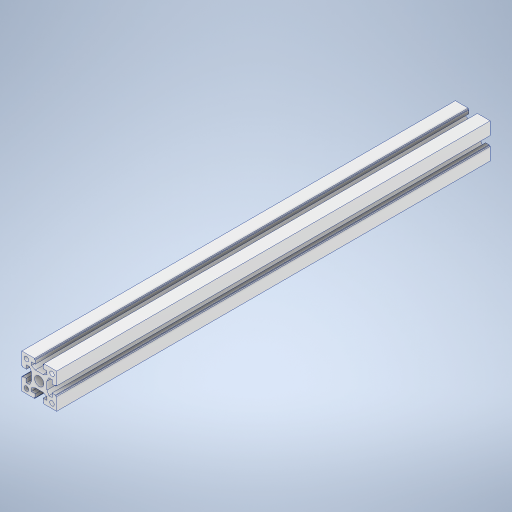
# Autodesk Inventor part: Union soporte P45X45 Trigger
Saved by Autodesk Inventor 2024.2 (Build 282272000, 272)
## iProperties
Created: 2026-07-03
Part Number: Union soporte P45X45 Trigger
Material: Aluminum 6061
Document SubType Name: Modeling
Designer: ja.restrepo1
Density: 2.7 g/cm^3
Appearance: Aluminum - Flat
Author: ja.restrepo1
Autodesk Inventor part; units mm, degrees
ref_plane "YZ Plane" through (0, 0, 0) normal (1, 0, 0) x (0, 1, 0)
ref_plane "XZ Plane" through (0, 0, 0) normal (0, 1, 0) x (-1, 0, 0)
ref_plane "XY Plane" through (0, 0, 0) normal (0, 0, 1) x (1, 0, 0)
sketch "Sketch1" plane through (0, 0, 0) normal (0, 0, 1) x (1, 0, 0)
  line L0 (-22.5, 22.5) -> (-6, 22.5)
  line L1 (-6, 22.5) -> (-6, 21)
  line L2 (-6, 21) -> (-5, 21)
  line L3 (-5, 21) -> (-5, 16.5)
  line L4 (-5, 16.5) -> (-10, 16.5)
  line L5 (-10, 16.5) -> (-10, 12.5)
  line L6 (-10, 12.5) -> (-5, 10)
  line L7 (-5, 10) -> (5, 10)
  line L8 (10, 12.5) -> (10, 16.5)
  line L9 (10, 16.5) -> (5, 16.5)
  line L10 (5, 16.5) -> (5, 21)
  line L11 (5, 21) -> (6, 21)
  line L12 (6, 21) -> (6, 22.5)
  line L13 (6, 22.5) -> (22.5, 22.5)
  line L14 (22.5, 22.5) -> (22.5, 6)
  line L15 (22.5, 6) -> (21, 6)
  line L16 (21, 6) -> (21, 5)
  line L17 (21, 5) -> (16.5, 5)
  line L18 (10, 12.5) -> (5, 10)
  line L19 (-22.5, 0) -> (-22.5, 104.1484) construction
  line L20 (-22.5, 0) -> (77.4828, 0) construction
  line L21 (16.5, 5) -> (16.5, 10)
  line L22 (16.5, 10) -> (12.5, 10)
  line L23 (12.5, 10) -> (10, 5)
  line L24 (10, 5) -> (10, 0)
  circle A0 centre (0, 0) radius 6
  circle A1 centre (16.5, 16.5) radius 3
  line L25 (-22.5, 0) -> (45.512, 0) construction
  line L26 (21, -6) -> (21, -5)
  line L27 (22.5, -6) -> (21, -6)
  line L28 (10, -12.5) -> (10, -16.5)
  line L29 (12.5, -10) -> (10, -5)
  line L30 (16.5, -5) -> (16.5, -10)
  line L31 (16.5, -10) -> (12.5, -10)
  line L32 (10, -12.5) -> (5, -10)
  line L33 (22.5, -22.5) -> (22.5, -6)
  circle A2 centre (16.5, -16.5) radius 3
  line L34 (6, -22.5) -> (22.5, -22.5)
  line L35 (5, -16.5) -> (5, -21)
  line L36 (5, -21) -> (6, -21)
  line L37 (6, -21) -> (6, -22.5)
  line L38 (10, -16.5) -> (5, -16.5)
  line L39 (21, -5) -> (16.5, -5)
  line L40 (10, -5) -> (10, 0)
  line L41 (-5, -10) -> (5, -10)
  line L42 (-22.5, -22.5) -> (-6, -22.5)
  line L43 (-6, -22.5) -> (-6, -21)
  line L44 (-6, -21) -> (-5, -21)
  line L45 (-5, -21) -> (-5, -16.5)
  line L46 (-5, -16.5) -> (-10, -16.5)
  line L47 (-10, -16.5) -> (-10, -12.5)
  line L48 (-10, -12.5) -> (-5, -10)
  line L49 (-22.5, -22.5) -> (-22.5, 22.5)
  line L50 (0, -24.7031) -> (0, 16.5) construction
  line L51 (-12.5, 10) -> (-10, 5)
  line L52 (-16.5, 10) -> (-12.5, 10)
  line L53 (-16.5, 5) -> (-16.5, 10)
  line L54 (-21, 5) -> (-16.5, 5)
  line L55 (-21, 6) -> (-21, 5)
  line L56 (-22.5, 6) -> (-21, 6)
  line L57 (-10, 5) -> (-10, 0)
  line L58 (-10, -5) -> (-10, 0)
  line L59 (-12.5, -10) -> (-10, -5)
  line L60 (-16.5, -10) -> (-12.5, -10)
  line L61 (-16.5, -5) -> (-16.5, -10)
  line L62 (-21, -5) -> (-16.5, -5)
  line L63 (-21, -6) -> (-21, -5)
  line L64 (-22.5, -6) -> (-21, -6)
  circle A3 centre (-16.5, 16.5) radius 3
  circle A4 centre (-16.5, -16.5) radius 3
  point P0 (0, 10)
  point P1 (0, -10)
  point P2 (-69.7014, -56.3955)
  point P3 (-69.7014, -68.3955)
  point P4 (-36.78, -20.9511)
  point P5 (-36.78, -32.9511)
  dimension "d0" = 22.5
  dimension "d1" = 20
  dimension "d2" = 1.5
  dimension "d3" = 1.5
  dimension "d4" = 10
  dimension "d5" = 12
  dimension "d6" = 12.5
  dimension "d7" = 22.5
  dimension "d8" = 5
  dimension "d9" = 6
  dimension "d10" = 10
  dimension "d11" = 6
  dimension "d12" = 4
  dimension "d13" = 5
  dimension "d14" = 6
  dimension "d15" = 45
  dimension "d16" = 10
  dimension "d17" = 4
  dimension "d18" = 12.5
  dimension "d19" = 6
  dimension "d20" = 12
  dimension "d21" = 22.5
  dimension "d22" = 6
  dimension "d23" = 39
  dimension "d24" = 16.5
  dimension "d25" = 12.5
  constraints: 130 end point, 42 symmetric about line, 13 point on line, 12 perpendicular, 6 coincident, 5 centre point, 4 vertical, 3 horizontal alignment, 2 collinear, 2 horizontal, 2 midpoint, 2 parallel, 1 vertical alignment, 3 other
  measures "d0" distance from line of point (-22.5, 0) L0
  measures "d1" distance between parallel lines of L5 L8
  measures "d2" distance between parallel lines of L0 L2
  measures "d3" distance between parallel lines of L14 L16
  measures "d4" distance between parallel lines of L10 L3
  measures "d5" distance between parallel lines of L1 L12
  measures "d6" distance between parallel lines of L0 L7
  measures "d7" horizontal distance of point (0, 10) point (-22.5, 0)
  measures "d8" distance from line of point (0, 10) L10
  measures "d9" distance from line of point (0, 10) L12
  measures "d10" distance from line of point (0, 10) L5
  measures "d11" distance between parallel lines of L0 L4
  measures "d12" distance of L4.end L5.end
  measures "d13" distance between parallel lines of L20 L17
  measures "d14" distance between parallel lines of L20 L15
  measures "d15" distance from line of point (-22.5, 0) L14
  measures "d16" distance between parallel lines of L20 L22
  measures "d17" distance of L21.end L22.end
  measures "d18" distance between parallel lines of L14 L24
  measures "d19" distance between parallel lines of L14 L21
  measures "d20" diameter of A0
  measures "d21" distance of point (-22.5, 0) A0.centre
  measures "d22" diameter of A1
  measures "d23" horizontal distance of A1.centre point (-22.5, 0)
  measures "d24" vertical distance of point (-22.5, 0) A1.centre
  measures "d25" distance from line of point (-22.5, 0) L57
extrude "Extrusion1" add sketch "Sketch1" along normal mid plane 560 contours L0 L1 L2 L3 L4 L5 L6 L7 L18 L8 L9 L10 L11 L12 L13 L14 L15 L16 L17 L21 L22 L23 L24 L40 L29 L31 L30 L39 L26 L27 L33 L34 L37 L36 L35 L38 L28 L32 L41 L48 L47 L46 L45 L44 L43 L42 L49 L64 L63 L62 L61 L60 L59 L58 L57 L51 L52 L53 L54 L55 L56
equation "\"d3\" = d2"
equation "\"d8\" = 0.5 * d4"
equation "\"d9\" = 0.5 * d5"
equation "\"d10\" = 0.5 * d1"
equation "\"d13\" = d8"
equation "\"d14\" = d9"
equation "\"d16\" = d10"
equation "\"d17\" = d12"
equation "\"d19\" = d11"
body "Solid1"
